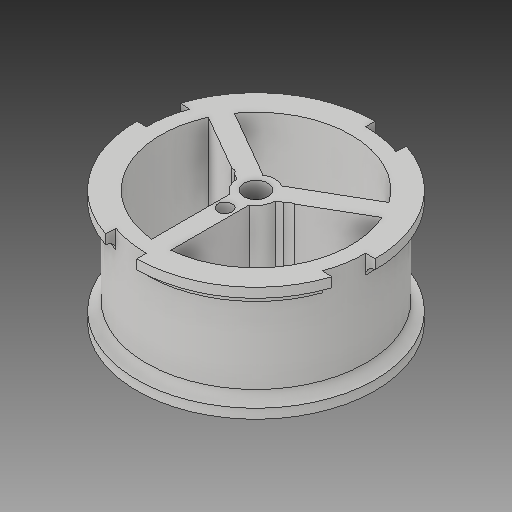
# Autodesk Inventor part: Wheel
Saved by Autodesk Inventor 2018 (Build 220112000, 112)
## iProperties
Created: 2019-03-25
Part Number: Wheel
Material: Типовые
Document SubType Name: Modeling
Designer: cosko
Density: 1 g/cm^3
Appearance: По умолчанию
Mass: 16.7421 g
Surface Area: 120.92 cm^2
Volume: 16.7421 cm^3
Author: cosko
Autodesk Inventor part; units mm, degrees
ref_plane "YZ Plane" through (0, 0, 0) normal (1, 0, 0) x (0, 1, 0)
ref_plane "XZ Plane" through (0, 0, 0) normal (0, 1, 0) x (-1, 0, 0)
ref_plane "XY Plane" through (0, 0, 0) normal (0, 0, 1) x (1, 0, 0)
sketch "Эскиз1" plane through (0, 0, 0) normal (0, 0, 1) x (1, 0, 0)
  line L0 (0, 0) -> (20, 0) construction
  line L1 (20, 0) -> (20, 12) construction
  line L2 (20, 12) -> (20, -12)
  line L3 (20, 12) -> (25, 12)
  line L4 (25, 12) -> (25, -12)
  line L5 (25, -12) -> (20, -12)
  line L6 (20, -12) -> (20, 12)
  line L7 (25, 12) -> (20, 12) construction
  line L8 (20, 12) -> (20, 10) construction
  line L9 (25, 10) -> (25, 10) construction
  line L10 (25, 10) -> (25, 12) construction
  line L11 (25, -12) -> (20, -12) construction
  line L12 (20, -12) -> (20, -10) construction
  line L13 (20, -10) -> (25, -10) construction
  line L14 (25, -10) -> (25, -12) construction
  line L15 (25, -10) -> (25, -10)
  line L16 (23, -8) -> (23, 8)
  line L17 (25, 10) -> (25, -10)
  arc A0 (25, 10) -> (23, 8) centre (25, 8) ccw
  arc A1 (23, -8) -> (25, -10) centre (25, -8) ccw
  arc A2 (25, 10) -> (23, 8) centre (25, 8) ccw
  line L18 (23, 8) -> (23, -8)
  arc A3 (23, -8) -> (25, -10) centre (25, -8) ccw
  line L19 (25, -10) -> (25, 10)
  line L20 (0, 0) -> (0, 12)
  dimension "d0" = 20
  dimension "d1" = 12
  dimension "d2" = 24
  dimension "d3" = 5
  dimension "d4" = 2
  dimension "d5" = 2
  dimension "d7" = 2
  constraints: 42 end point, 8 point on circle, 8 tangent, 7 parallel, 5 horizontal, 4 centre point, 4 perpendicular, 3 point on line, 3 vertical, 1 collinear, 1 equal radius
  measures "d0" distance of L0.start L0.end
  measures "d1" distance of L0.end L1.end
  measures "d2" distance of L1.end L2.end
  measures "d3" distance of L4.end L5.end
  measures "d4" distance of L8.end L7.end
  measures "d5" distance of L11.end L12.end
  measures "d7" radius of A0
revolve "Вращение1" add sketch "Эскиз1" angle 360 about axis through (0, 0, 0) along (0, 1, 0) contours L3 L4 A0 L16 A1 L5 L2
sketch "Эскиз2" plane through (0, -12, 0) normal (0, -1, 0) x (1, 0, 0)
  circle A0 centre (0, 0) radius 10
  circle A1 centre (0, 0) radius 2.5
  line L0 (0, 0) -> (0, -5) construction
  line L1 (0, -5) -> (0, 5) construction
  line L2 (0, 5) -> (0, 8) construction
  circle A2 centre (0, 6.5) radius 1.5
  circle A3 centre (-6.5, 0) radius 1.5
  circle A4 centre (0, -6.5) radius 1.5
  circle A5 centre (6.5, 0) radius 1.5
  point P0 (-8, 0)
  point P1 (0, -8)
  point P2 (8, 0)
  dimension "d9" = 20
  dimension "d10" = 5
  dimension "d11" = 5
  dimension "d12" = 10
  dimension "d13" = 3
  dimension "d16" = 360
  constraints: 6 end point, 2 centre point, 2 coincident, 2 horizontal alignment, 2 vertical, 2 vertical alignment, 1 midpoint, 1 point on line, 21 other
  measures "d9" diameter of A0
  measures "d10" diameter of A1
  measures "d11" distance of L0.start L0.end
  measures "d12" distance of L0.end L1.end
  measures "d13" distance of L1.end L2.end
extrude "Выдавливание1" add sketch "Эскиз2" against normal blind 3
sketch "Эскиз3" plane through (0, -12, 0) normal (0, -1, 0) x (1, 0, 0)
  circle A0 centre (0, 0) radius 10 construction
  circle A1 centre (0, 0) radius 20 construction
  line L0 (2, 19.899749) -> (2, 9.797959)
  line L1 (-2, 9.797959) -> (-2, 19.899749)
  arc A2 (2, 19.899749) -> (-2, 19.899749) centre (0, 0) ccw
  line L2 (1.558389, 9.797959) -> (2, 9.797959)
  line L3 (2, 9.797959) -> (2, 1.685342)
  line L4 (-2, 1.685342) -> (-2, 9.797959)
  line L5 (1.533287, 9.881752) -> (1.846516, 8.836167) construction
  arc A3 (2, 1.685342) -> (-2, 1.685342) centre (0, -0.362348) ccw
  line L6 (-18.233688, -8.217824) -> (-9.485281, -3.166929)
  line L7 (-7.485281, -6.63103) -> (-16.233688, -11.681925)
  arc A4 (-18.233688, -8.217824) -> (-16.233688, -11.681925) centre (0, 0) ccw
  line L8 (-0.459549, -2.574722) -> (-7.485281, -6.63103)
  arc A5 (-2.459549, 0.88938) -> (-0.459549, -2.574722) centre (0.313802, 0.181174) ccw
  line L9 (-9.485281, -3.166929) -> (-2.459549, 0.88938)
  line L10 (16.233688, -11.681925) -> (7.485281, -6.63103)
  line L11 (9.485281, -3.166929) -> (18.233688, -8.217824)
  arc A6 (16.233688, -11.681925) -> (18.233688, -8.217824) centre (0, 0) ccw
  line L12 (2.459549, 0.88938) -> (9.485281, -3.166929)
  arc A7 (0.459549, -2.574722) -> (2.459549, 0.88938) centre (-0.313802, 0.181174) ccw
  line L13 (7.485281, -6.63103) -> (0.459549, -2.574722)
  dimension "d23" = 360
  constraints: 28 end point, 17 point on circle, 6 centre point, 2 parallel, 1 horizontal, 1 perpendicular, 1 point on line, 43 other
sketch "Эскиз4" plane through (0, -9, 0) normal (0, 1, 0) x (1, 0, 0)
  circle A0 centre (0, 0) radius 2.5
  circle A1 centre (0, 0) radius 4
  dimension "d25" = 8
  constraints: 2 centre point, 2 coincident
  measures "d25" diameter of A1
extrude "Выдавливание2" add sketch "Эскиз4" along normal up to surface (21 mm away)
extrude "Выдавливание3" add sketch "Эскиз3" against normal blind 24
sketch "Эскиз5" plane through (0, -12, 0) normal (0, -1, 0) x (1, 0, 0)
  circle A0 centre (0, -6.5) radius 1.5 projected
  circle A1 centre (0, -6.5) radius 1.5
  circle A2 centre (0, 0) radius 2.5 construction
  circle A3 centre (6.5, 0) radius 1.5
  circle A4 centre (0, 6.5) radius 1.5
  circle A5 centre (-6.5, 0) radius 1.5
  dimension "d32" = 360
  constraints: 5 centre point, 2 coincident, 1 concentric, 9 other
extrude "Выдавливание4" cut sketch "Эскиз5" against normal blind 24
sketch "Эскиз8" plane through (0, 12, 0) normal (0, 1, 0) x (1, 0, 0)
  circle A0 centre (0, 0) radius 23
  circle A1 centre (0, 0) radius 23
  line L0 (0, -23) -> (0, -25.980192)
  line L1 (0, -25.980192) -> (-7.917544, -25.604358)
  line L2 (-7.917544, -25.604358) -> (-7.730405, -21.661968)
  circle A2 centre (0, 0) radius 23
  arc A3 (-7.730405, -21.661968) -> (0, -23) centre (0, 0) ccw
  line L3 (23, 0) -> (25.980192, 0)
  line L4 (25.980192, 0) -> (25.604358, -7.917544)
  line L5 (25.604358, -7.917544) -> (21.661968, -7.730405)
  arc A4 (21.661968, -7.730405) -> (23, 0) centre (0, 0) ccw
  line L6 (0, 23) -> (0, 25.980192)
  line L7 (0, 25.980192) -> (7.917544, 25.604358)
  line L8 (7.917544, 25.604358) -> (7.730405, 21.661968)
  arc A5 (7.730405, 21.661968) -> (0, 23) centre (0, 0) ccw
  line L9 (-23, 0) -> (-25.980192, 0)
  line L10 (-25.980192, 0) -> (-25.604358, 7.917544)
  line L11 (-25.604358, 7.917544) -> (-21.661968, 7.730405)
  arc A6 (-21.661968, 7.730405) -> (-23, 0) centre (0, 0) ccw
  dimension "d42" = 360
  constraints: 24 end point, 9 point on circle, 4 centre point, 1 concentric, 1 perpendicular, 1 vertical, 1 vertical alignment, 38 other
extrude "Выдавливание5" cut sketch "Эскиз8" against normal blind 10 contours L3 L4 L5 A0 | A0 L6 L7 L8 | L0 L1 L2 A0 | A0 L9 L10 L11
